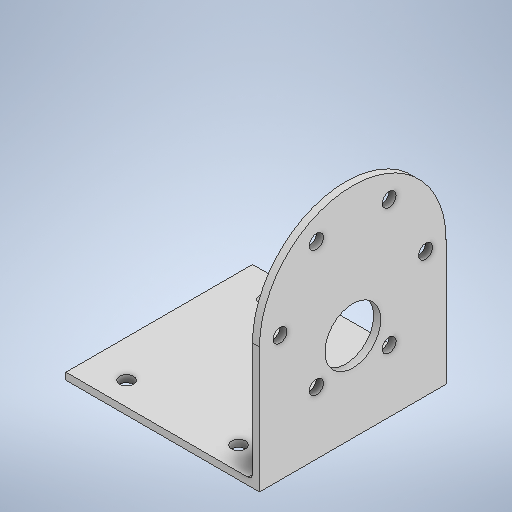
# Autodesk Inventor part: motor_support
Saved by Autodesk Inventor 2025 (Build 290162010, 162A)
## iProperties
Created: 2024-10-24
Part Number: motor_support
Material: Generic
Document SubType Name: Modeling
Designer: fist5
Density: 1 g/cm^3
Appearance: Default
Author: fist5
Autodesk Inventor part; units mm, degrees
ref_plane "YZ Plane" through (0, 0, 0) normal (1, 0, 0) x (0, 1, 0)
ref_plane "XZ Plane" through (0, 0, 0) normal (0, 1, 0) x (-1, 0, 0)
ref_plane "XY Plane" through (0, 0, 0) normal (0, 0, 1) x (1, 0, 0)
sketch "Sketch1" plane through (0, 0, 0) normal (0, 1, 0) x (-1, 0, 0)
  line L0 (-20, 20) -> (-20, -20)
  line L1 (-20, -20) -> (20, -20)
  line L2 (20, -20) -> (20, 20)
  line L3 (20, 20) -> (-20, 20)
  line L4 (-20, 20) -> (20, -20) construction
  line L5 (-20, -20) -> (20, 20) construction
  point P0 (0, 0)
  point P1 (0, -20)
  dimension "d0" = 40
  dimension "d1" = 40
  constraints: 12 end point, 3 midpoint, 2 parallel, 1 perpendicular, 1 vertical
  measures "d0" distance from line of point (0, -20) L3
  measures "d1" distance between parallel lines of L0 L2
extrude "Extrusion1" add sketch "Sketch1" along normal blind 1.5
sketch "Sketch2" plane through (20, 0, 20) normal (1, 0, 0) x (0, 0, -1)
  circle A0 centre (20, 26.9) radius 20
  line L0 (40, 1.5) -> (40, 46.9)
  line L1 (40, 1.5) -> (0, 1.5) projected
  line L2 (0, 1.5) -> (0, 46.9)
  line L3 (0, 46.9) -> (40, 46.9)
  line L4 (0, 0) -> (40, 0) projected
  line L5 (0, 0) -> (0, 1.5) projected
  line L6 (0, 1.5) -> (0, 0)
  line L7 (40, 0) -> (0, 0) projected
  line L8 (0, 0) -> (40, 0)
  line L9 (40, 0) -> (40, 1.5) projected
  line L10 (40, 0) -> (40, 1.5)
  point P0 (20, 0)
  point P1 (40, 26.9)
  point P2 (0, 26.9)
  dimension "d4" = 45.4
  constraints: 12 end point, 3 tangent, 3 vertical, 2 equal length, 1 centre point, 1 perpendicular
  measures "d4" distance between parallel lines of L1 L3
extrude "Extrusion2" add sketch "Sketch2" along normal blind 1.5 contours A0 | L0 L1 L2 A0 | L9 L4 L5 L1
fillet "Fillet1" radius 1 1 edges at (20, 1.5, 0)
sketch "Sketch3" plane through (21.5, 0, 20) normal (1, 0, 0) x (0, 0, -1)
  arc A0 (40, 26.9) -> (0, 26.9) centre (20, 26.9) ccw projected
  circle A1 centre (20, 26.9) radius 15.605
  circle A2 centre (20, 19) radius 5.98
  circle A3 centre (4.395, 26.9) radius 1.5
  point P0 (20, 0)
  dimension "d8" = 31.21
  dimension "d9" = 7.9
  dimension "d10" = 11.96
  dimension "d11" = 3
  constraints: 2 centre point, 2 horizontal alignment, 1 coincident, 1 vertical alignment, 2 other
  measures "d9" distance of A2.centre point (20, 26.9)
  measures "d10" diameter of A2
  measures "d11" diameter of A3
extrude "Extrusion3" cut sketch "Sketch3" against normal up to surface (1.5 mm away) contours A2
extrude "Extrusion4" cut sketch "Sketch3" against normal up to surface (1.5 mm away) contours A3 A1 | A1 A3 picked at (4.9003, 26.9) picked at (3.9042, 26.9621)
pattern_circular "Circular Pattern1" count 6 over 360 about axis through (20, 26.9, 0) along (1, 0, 0) of "Extrusion4"
sketch "Sketch4" plane through (0, 1.5, 0) normal (0, 1, 0) x (1, 0, 0)
  line L0 (12, 15) -> (-12, 15)
  line L1 (-12, 15) -> (-12, -15)
  line L2 (-12, -15) -> (12, -15)
  line L3 (12, -15) -> (12, 15)
  line L4 (-20, 20) -> (-20, -20) projected
  line L5 (-20, -20) -> (19, -20) projected
  circle A0 centre (-12, 15) radius 1.5
  point P0 (0, 0)
  dimension "d19" = 30
  dimension "d20" = 24
  dimension "d21" = 8
  dimension "d22" = 5
  dimension "d23" = 3
  constraints: 8 end point, 2 parallel, 1 centre point, 1 coincident, 1 horizontal, 1 perpendicular
  measures "d19" distance between parallel lines of L2 L0
  measures "d20" distance between parallel lines of L1 L3
  measures "d21" distance between parallel lines of L4 L1
  measures "d22" distance between parallel lines of L5 L2
  measures "d23" diameter of A0
extrude "Extrusion5" cut sketch "Sketch4" against normal up to surface (1.5 mm away) contours A0 L1 L0 | L0 L1 A0
pattern_linear "Rectangular Pattern1" count 2 spacing 24 along (1, 0, 0) count 2 spacing 30 along (0, 0, 1) of "Extrusion5"
body "Solid1"
